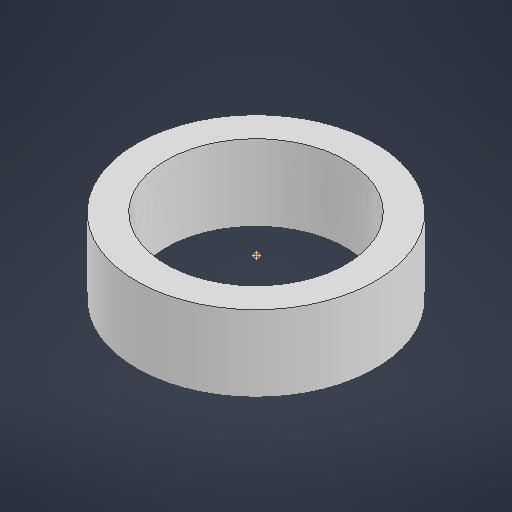
# Autodesk Inventor part: Outboard_Bearing_Housing
Saved by Autodesk Inventor 2026.1 (Build 301233000, 233)
## iProperties
Created: 2026-09-19
Part Number: Outboard_Bearing_Housing
Material: Generic
Document SubType Name: Modeling
Designer: share
Density: 1 g/cm^3
Appearance: Default
Author: share
Autodesk Inventor part; units mm, degrees
sketch "Sketch2" plane through (0, 0, 0) normal (0, 1, 0) x (-1, 0, 0)
  circle A0 centre (0, 0) radius 15.0812
  circle A1 centre (0, 0) radius 20
  dimension "d7" = 30.1625
  dimension "d8" = 40
  constraints: 2 centre point, 2 coincident
  measures "d7" diameter of A0
  measures "d8" diameter of A1
extrude "Extrusion2" add sketch "Sketch2" along normal mid plane 12.7
equation "\"Bearing_OD\" = 30.1625"
body "Solid2"
